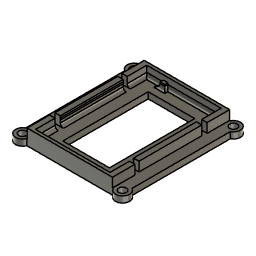
meanwell_holder v3 (Autodesk Fusion 360 design; units mm, degrees)
Autodesk Fusion 360 part; units mm, degrees
note: some values were not read from the file. Chosen so that the rebuilt part matches the saved one: which bodies a step acts on.
sketch "Sketch1" plane through (0, 0, 0) normal (0, 0, 1) x (1, 0, 0)
  line L0 (-23.5, 35.315) -> (23.5, 35.315)
  line L1 (23.5, 35.315) -> (23.5, -35.315)
  line L2 (23.5, -35.315) -> (-23.5, -35.315)
  line L3 (-23.5, -35.315) -> (-23.5, 35.315)
  line L4 (-23.5, 35.315) -> (23.5, -35.315) construction
  line L5 (23.5, 35.315) -> (-23.5, -35.315) construction
  circle A0 centre (-32, 35.75) radius 2.5
  circle A1 centre (32, 35.75) radius 2.5
  circle A2 centre (-31.9851, -36.25) radius 2.5
  circle A3 centre (32.0129, -35.7484) radius 2.5
  line L6 (-32, 35.75) -> (-30.3326, 33.8872) construction
  arc A4 (-34, -32.2263) -> (-27.7424, -37.75) centre (-31.9851, -36.25) ccw
  arc A5 (27.9826, -37.75) -> (34, -31.7109) centre (32.0129, -35.7484) ccw
  line L7 (-23.5, 26.2539) -> (28.9987, -32.397) construction
  arc A6 (34, 31.7189) -> (27.9689, 37.75) centre (32, 35.75) ccw
  line L8 (23.5, 26.2539) -> (-28.9987, -32.397) construction
  arc A7 (-27.9689, 37.75) -> (-34, 31.7189) centre (-32, 35.75) ccw
  line L9 (0, 35.75) -> (0, -35.75)
  line L10 (-34.0004, 29.5655) -> (-34.0155, -30.0752)
  line L11 (-25.6605, -37.75) -> (25.8288, -37.75)
  line L12 (34, -29.5596) -> (34, 29.5653)
  line L13 (25.8153, 37.75) -> (-25.8153, 37.75)
  line L14 (27.9689, 37.75) -> (-27.9689, 37.75)
  line L15 (25.8153, 37.75) -> (27.9689, 37.75)
  line L16 (34, 29.5653) -> (34, 31.7189)
  line L17 (34, -31.7109) -> (34, 31.7189)
  line L18 (-34, 31.7189) -> (-34, -32.2263)
  line L19 (-34, -37.7299) -> (-34, -37.75)
  line L20 (-34, -37.75) -> (-33.9851, -37.75)
  line L21 (-27.7424, -37.75) -> (27.9826, -37.75)
  dimension "d1" = 47
  dimension "d2" = 70.63
  dimension "d3" = 64
  dimension "d5" = 5
  dimension "d6" = 5
  dimension "d7" = 5
  dimension "d8" = 5
  dimension "d9" = 9
  dimension "d10" = 9
  dimension "d11" = 9
  dimension "d12" = 9
  dimension "d13" = 71.5
  constraint horizontal L0
  constraint perpendicular L0 L1
  constraint parallel L0 L2
  constraint parallel L1 L3
  constraint coincident L4 origin
  constraint coincident L5 origin
  constraint coincident origin L6
  constraint coincident A0.centre L6.start
  constraint concentric A1 A6
  constraint concentric A3 A5
  constraint concentric A2 A4
  constraint coincident A0 L6.end
  constraint collinear L6 L7
  constraint coincident L3 L7.start
  constraint coincident L1 L8.start
  constraint midpoint origin L9
  constraint horizontal L15
  constraint perpendicular L15 L16
  constraint horizontal L20
  constraint coincident A4.end L20
  constraint collinear L18 L19
  constraint coincident A2 L19.start
  constraint coincident A2 L20.end
  constraint collinear L20 L21
  measures "d1" distance of L1.end L2.end
  measures "d2" distance of L0.end L1.end
  measures "d3" distance of A2.centre A3.centre
  measures "d5" diameter of A0
  measures "d6" diameter of A1
  measures "d7" diameter of A2
  measures "d8" diameter of A3
  measures "d9" diameter of A6
  measures "d10" diameter of A5
  measures "d11" diameter of A4
  measures "d12" diameter of A7
  measures "d13" distance of L9.start L9.end
extrude "Extrude1" add sketch "Sketch1" along normal blind 4 contours L0 L2 L3 L9 | L0 L1 L2 L9 | A4 A5 A6 A7 L11 L12 L13 L14 L15 L16 L17 L18 L21 makes body 1
sketch "Sketch2" plane through (0, 0, 4) normal (0, 0, 1) x (-1, 0, 0)
  circle A0 centre (-32, -35.75) radius 2.5
  circle A1 centre (-32.0129, 35.7484) radius 2.5
  line L0 (33.9851, 37.75) -> (34, 37.75)
  line L1 (34, 37.75) -> (34, 37.7299)
  arc A2 (33.9851, 37.75) -> (34, 37.7299) centre (31.9851, 36.25) ccw
  circle A3 centre (32, -35.75) radius 2.5
  line L2 (-27.9689, -37.75) -> (27.9689, -37.75)
  arc A4 (27.9689, -37.75) -> (34, -31.7189) centre (32, -35.75) ccw
  line L3 (34, -31.7189) -> (34, 32.2263)
  arc A5 (34, 32.2263) -> (27.7424, 37.75) centre (31.9851, 36.25) ccw
  line L4 (27.7424, 37.75) -> (-27.9826, 37.75)
  arc A6 (-27.9826, 37.75) -> (-34, 31.7109) centre (-32.0129, 35.7484) ccw
  line L5 (-34, 31.7109) -> (-34, -31.7189)
  arc A7 (-34, -31.7189) -> (-27.9689, -37.75) centre (-32, -35.75) ccw
  line L6 (23.5, -35.315) -> (-23.5, -35.315)
  line L7 (23.5, 35.315) -> (23.5, -35.315)
  line L8 (-23.5, -35.315) -> (-23.5, 35.315)
  line L9 (-23.5, 35.315) -> (23.5, 35.315)
  line L10 (24, 32.815) -> (24, -35.815)
  line L11 (-25.5, 37.315) -> (25.5, 37.315)
  line L12 (25.5, 37.315) -> (25.5, -37.315)
  line L13 (25.5, -37.315) -> (-25.5, -37.315)
  line L14 (-25.5, -37.315) -> (-25.5, 37.315)
  line L15 (21, 35.815) -> (24, 32.815)
  line L16 (-21, 35.815) -> (-24, 32.815)
  line L17 (23.5, 35.315) -> (8.8, 35.315)
  line L18 (5.8, 33.815) -> (8.8, 33.815)
  line L19 (8.8, 33.815) -> (8.8, 35.815)
  line L20 (5.8, 36.815) -> (5.8, 33.815)
  line L21 (-8, 33.815) -> (-5, 33.815)
  line L22 (-5, 33.815) -> (-5, 35.815)
  line L23 (-8, 35.815) -> (-8, 33.815)
  line L24 (8.8, 35.815) -> (21, 35.815)
  line L25 (-21, 35.815) -> (-7, 35.815)
  line L26 (-5, 35.815) -> (6.8, 35.815)
  line L27 (23.5, 35.315) -> (8.8, 35.315)
  line L28 (5.8, 35.315) -> (-5, 35.315)
  line L29 (-21, -35.815) -> (-24, -32.815)
  line L30 (-23.5, -35.315) -> (10.4, -35.315)
  line L31 (13.4, -35.815) -> (13.4, -33.815)
  line L32 (13.4, -33.815) -> (10.4, -33.815)
  line L33 (10.4, -33.815) -> (10.4, -35.815)
  line L34 (10.4, -35.815) -> (-21, -35.815)
  line L35 (24, -35.815) -> (13.4, -35.815)
  line L36 (-23.5, -35.315) -> (-23.5, -15.615)
  line L37 (-22, -15.615) -> (-24, -15.615)
  line L38 (-24, -12.615) -> (-22, -12.615)
  line L39 (-22, -12.615) -> (-22, -15.615)
  line L40 (-24, -32.815) -> (-24, -15.615)
  line L41 (-24, -12.615) -> (-24, 32.815)
  line L42 (25.5, -37.75) -> (-25.5, -37.75)
  line L43 (-25.5, -37.75) -> (-25.5, 37.75)
  line L44 (-25.5, 37.75) -> (25.5, 37.75)
  line L45 (25.5, 37.75) -> (25.5, -37.75)
  point P0 (-24, 35.815)
  point P1 (24, 35.815)
  point P2 (-24, -35.815)
  point P3 (7.3, 35.315)
  point P4 (-6.5, 35.315)
  point P5 (-23.5, -14.115)
  dimension "d20" = -2
  dimension "d21" = 3
  dimension "d22" = 3
  dimension "d23" = 3
  dimension "d24" = 3
  dimension "d25" = 16.2
  dimension "d26" = 30
  dimension "d31" = 3
  dimension "d32" = 3
  dimension "d34" = 3
  dimension "d36" = 21.2
  constraint coincident P1 L25
  constraint coincident P1 L10
  constraint coincident P0 L25
  constraint coincident P0 L40
  constraint coincident L7.start L9.end
  constraint perpendicular L7 L17
  constraint perpendicular L7 L27
  constraint horizontal L18
  constraint perpendicular L18 L19
  constraint parallel L19 L20
  constraint horizontal L21
  constraint perpendicular L21 L22
  constraint parallel L22 L23
  constraint coincident L19.end L25
  constraint collinear L24 L25
  constraint coincident L22.end L25
  constraint coincident L23.start L25
  constraint collinear L25 L26
  constraint coincident L22 L28.end
  constraint coincident L20 L28.start
  constraint collinear L27 L28
  constraint coincident L19 L17.end
  constraint coincident P2 L35
  constraint coincident P2 L40
  constraint coincident L6.end L8.start
  constraint perpendicular L12 L30
  constraint parallel L31 L33
  constraint coincident L33.end L35
  constraint collinear L34 L35
  constraint coincident L33 L30.end
  constraint perpendicular L30 L36
  constraint horizontal L37
  constraint parallel L37 L38
  constraint coincident L38.start L40
  constraint collinear L40 L41
  constraint coincident L37 L36.end
  constraint horizontal L42
  constraint vertical L43
  constraint horizontal L44
  constraint vertical L45
  constraint coincident L4 L43.end
  constraint coincident L2 L42.start
  measures "d21" distance of P1 L15.start
  measures "d22" distance of P1 L10.start
  measures "d23" distance of P0 L16.start
  measures "d24" distance of P0 L16.end
  measures "d25" distance of L7.start P3
  measures "d26" distance of L7.start P4
  measures "d31" distance of P2 L29.start
  measures "d32" distance of P2 L29.end
  measures "d34" distance of L31.end L32.end
  measures "d36" distance of L6.end P5
extrude "Extrude2" add sketch "Sketch2" along normal blind 3 contours L2 L13 L42 L43 L45 | L11 L12 L13 L14 L43 L45 | L4 L11 L43 L44 L45 | L6 L31 L32 L33 | L7 L9 L15 L17 L27 | L6 L8 L29 L30 L36 | L9 L18 L19 L20 | L8 L37 L38 L39 | L9 L21 L22 L23 | L8 L9 L16 bodies 1
sketch "Sketch3" plane through (0, 0, 7) normal (0, 0, 1) x (-1, 0, 0)
  line L0 (-22, -15.615) -> (-22, -12.615)
  line L1 (-22, -12.615) -> (-24, -12.615)
  line L2 (-24, -12.615) -> (-24, 32.815)
  line L3 (-24, 32.815) -> (-21, 35.815)
  line L4 (-21, 35.815) -> (-8, 35.815)
  line L5 (-8, 35.815) -> (-8, 33.815)
  line L6 (-8, 33.815) -> (-5, 33.815)
  line L7 (-5, 33.815) -> (-5, 35.815)
  line L8 (-5, 35.815) -> (5.8, 35.815)
  line L9 (5.8, 35.815) -> (5.8, 33.815)
  line L10 (5.8, 33.815) -> (8.8, 33.815)
  line L11 (8.8, 33.815) -> (8.8, 35.815)
  line L12 (8.8, 35.815) -> (21, 35.815)
  line L13 (21, 35.815) -> (24, 32.815)
  line L14 (24, 32.815) -> (24, -35.815)
  line L15 (24, -35.815) -> (13.4, -35.815)
  line L16 (13.4, -35.815) -> (13.4, -33.815)
  line L17 (13.4, -33.815) -> (10.4, -33.815)
  line L18 (10.4, -33.815) -> (10.4, -35.815)
  line L19 (10.4, -35.815) -> (-21, -35.815)
  line L20 (-21, -35.815) -> (-24, -32.815)
  line L21 (-24, -32.815) -> (-24, -15.615)
  line L22 (-24, -15.615) -> (-22, -15.615)
  line L23 (25.5, 37.75) -> (-25.5, 37.75)
  line L24 (-25.5, 37.75) -> (-25.5, -37.75)
  line L25 (-25.5, -37.75) -> (25.5, -37.75)
  line L26 (25.5, -37.75) -> (25.5, 37.75)
  line L27 (23.5, -35.315) -> (-23.5, -35.315)
  line L28 (23.5, 35.315) -> (23.5, -35.315)
  line L29 (-23.5, -35.315) -> (-23.5, 35.315)
  line L30 (-23.5, 35.315) -> (23.5, 35.315)
  line L31 (-24, 35.815) -> (24, 35.815)
  line L32 (24, 35.815) -> (24, -35.815)
  line L33 (24, -35.815) -> (-24, -35.815)
  line L34 (-24, -35.815) -> (-24, 35.815)
  dimension "d41" = -0.5
extrude "Extrude3" add sketch "Sketch3" along normal blind 3 bodies 1
sketch "Sketch4" plane through (0, -35.815, 0) normal (0, 1, 0) x (-1, 0, 0)
  line L0 (-21, 4) -> (-8, 4)
  line L1 (-8, 4) -> (-8, 7)
  line L2 (-8, 7) -> (-5, 7)
  line L3 (-5, 7) -> (-5, 4)
  line L4 (-5, 4) -> (5.8, 4)
  line L5 (5.8, 4) -> (5.8, 7)
  line L6 (5.8, 7) -> (8.8, 7)
  line L7 (8.8, 7) -> (8.8, 4)
  line L8 (8.8, 4) -> (21, 4)
  line L9 (21, 4) -> (21, 7)
  line L10 (21, 7) -> (24, 7)
  line L11 (24, 7) -> (24, 10)
  line L12 (24, 10) -> (-24, 10)
  line L13 (-24, 10) -> (-24, 7)
  line L14 (-24, 7) -> (-21, 7)
  line L15 (-21, 7) -> (-21, 4)
  line L16 (-24, 7) -> (-24, 7.6962)
  line L17 (-23.5981, 9.1962) -> (-22.4613, 11.1651)
  line L18 (-24, 8.5) -> (-20.9226, 8.5) construction
  line L19 (-24, 10) -> (-22.2313, 6.9366)
  line L20 (-24, 10) -> (-20.4627, 10) construction
  line L21 (-24, 10) -> (24, 10)
  line L22 (0, 10) -> (0, 2)
  arc A0 (-23.5981, 9.1962) -> (-24, 7.6962) centre (-21, 7.6962) ccw
  line L23 (-24, 10) -> (-24, 7)
  line L24 (24, 10) -> (24, 7)
  line L25 (24, 10) -> (22.2313, 6.9366)
  arc A1 (24, 7.6962) -> (23.5981, 9.1962) centre (21, 7.6962) ccw
  line L26 (23.5981, 9.1962) -> (22.4613, 11.1651)
  dimension "d44" = 1.5
  dimension "d45" = 60
  dimension "d46" = 60
  dimension "d47" = 3
  constraint coincident L13.end L14.start
  constraint coincident L13 L18.start
  constraint horizontal L18
  constraint horizontal L20
  constraint coincident L12.end L13.start
  constraint coincident L11.end L12.start
  constraint midpoint L21 L22.start
  constraint perpendicular L21 L22
  constraint coincident L18.start L17
  constraint coincident L18.start L16
  constraint tangent L17 A0
  constraint tangent L16 A0
  constraint symmetric L13.end L22 L10.end
  constraint symmetric L17.end L22 L26.end
  constraint symmetric L12.end L22 L11.end
  constraint symmetric L19.end L22 L25.end
  constraint symmetric L22 L17.start A1.end
  constraint symmetric L22 L16.end A1.start
  constraint symmetric L22 A0 A1
  constraint symmetric L22 L12.end L11.end
  measures "d44" distance of L13.end L18.start
  measures "d45" angle of L17 L18
  measures "d46" angle of L19 L20
  measures "d47" radius of A0
fillet "Fillet1" radius 2 1 faces at (0.9333, 4.205, 4) on bodies 1
extrude "Extrude7" add 1 faces at (25.5, -12.5833, 8) along direction (1, 0, 0) blind 2 on bodies 1 bodies 1
extrude "Extrude8" add 1 faces at (-25.5, 12.5833, 8) along direction (-1, 0, 0) blind 2 on bodies 1 bodies 1
sketch "Sketch5" plane through (0, 0, 4) normal (0, 0, 1) x (-1, 0, 0)
  line L0 (-27.5, 37.75) -> (-27.9826, 37.75)
  arc A0 (-27.9826, 37.75) -> (-34, 31.7109) centre (-32.0129, 35.7484) ccw
  line L1 (-34, 31.7109) -> (-34, -31.7189)
  arc A1 (-34, -31.7189) -> (-27.9689, -37.75) centre (-32, -35.75) ccw
  line L2 (-27.9689, -37.75) -> (-27.5, -37.75)
  circle A2 centre (-32.0129, 35.7484) radius 2.5
  circle A3 centre (-32, -35.75) radius 2.5
  line L3 (-38.0756, 37.75) -> (39, 37.75)
  line L4 (39, 37.75) -> (39, 34.75)
  line L5 (39, 34.75) -> (-38.0756, 34.75)
  line L6 (-38.0756, 34.75) -> (-38.0756, 37.75)
  line L7 (39, 20.25) -> (-38.0756, 20.25)
  line L8 (-38.0756, 23.25) -> (39, 23.25)
  line L9 (-38.0756, 20.25) -> (-38.0756, 23.25)
  line L10 (39, 23.25) -> (39, 20.25)
  line L11 (39, 5.75) -> (-38.0756, 5.75)
  line L12 (-38.0756, 8.75) -> (39, 8.75)
  line L13 (-38.0756, 5.75) -> (-38.0756, 8.75)
  line L14 (39, 8.75) -> (39, 5.75)
  line L15 (39, -8.75) -> (-38.0756, -8.75)
  line L16 (-38.0756, -5.75) -> (39, -5.75)
  line L17 (-38.0756, -8.75) -> (-38.0756, -5.75)
  line L18 (39, -5.75) -> (39, -8.75)
  line L19 (39, -23.25) -> (-38.0756, -23.25)
  line L20 (-38.0756, -20.25) -> (39, -20.25)
  line L21 (-38.0756, -23.25) -> (-38.0756, -20.25)
  line L22 (39, -20.25) -> (39, -23.25)
  line L23 (39, -37.75) -> (-38.0756, -37.75)
  line L24 (-38.0756, -34.75) -> (39, -34.75)
  line L25 (-38.0756, -37.75) -> (-38.0756, -34.75)
  line L26 (39, -34.75) -> (39, -37.75)
  line L27 (-27.5, -37.75) -> (-27.5, 37.75)
  dimension "d54" = 3
  dimension "d57" = 0
  dimension "d58" = -72.5
  constraint horizontal L3
  constraint vertical L4
  constraint horizontal L5
  constraint vertical L6
  measures "d54" distance of L3.start L5.end
extrude "Extrude5" cut sketch "Sketch5" along normal blind 32.11 contours L1 L7 L8 L27 | L7 L8 L10 L27 | L1 L19 L20 L27 | L19 L20 L22 L27 bodies 1
sketch "Sketch6" plane through (0, 0, 4) normal (0, 0, 1) x (-1, 0, 0)
  line L0 (-27.5, 20.25) -> (-22, 20.25)
  line L1 (-22, -20.25) -> (-27.5, -20.25)
  line L2 (-27.5, 37.75) -> (-27.9826, 37.75)
  arc A0 (-27.9826, 37.75) -> (-34, 31.7109) centre (-32.0129, 35.7484) ccw
  line L3 (-34, 31.7109) -> (-34, -31.7189)
  arc A1 (-34, -31.7189) -> (-27.9689, -37.75) centre (-32, -35.75) ccw
  line L4 (-27.9689, -37.75) -> (-27.5, -37.75)
  line L5 (-27.5, -23.25) -> (-22, -23.25)
  line L6 (-22, -23.25) -> (-22, -31.9866)
  line L7 (-22, -31.9866) -> (-20.1716, -33.815)
  line L8 (-20.1716, -33.815) -> (8.4, -33.815)
  line L9 (8.4, -33.815) -> (8.4, -31.815)
  line L10 (8.4, -31.815) -> (15.4, -31.815)
  line L11 (15.4, -31.815) -> (15.4, -33.815)
  line L12 (15.4, -33.815) -> (22, -33.815)
  line L13 (22, -33.815) -> (22, -23.25)
  arc A2 (27.9689, -37.75) -> (34, -31.7189) centre (32, -35.75) ccw
  line L14 (34, -31.7189) -> (34, 32.2263)
  arc A3 (34, 32.2263) -> (27.7424, 37.75) centre (31.9851, 36.25) ccw
  line L15 (27.7424, 37.75) -> (27.5, 37.75)
  line L16 (27.5, 23.25) -> (22, 23.25)
  line L17 (22, 23.25) -> (22, 31.9866)
  line L18 (22, 31.9866) -> (20.1716, 33.815)
  line L19 (20.1716, 33.815) -> (10.8, 33.815)
  line L20 (10.8, 33.815) -> (10.8, 31.815)
  line L21 (10.8, 31.815) -> (3.8, 31.815)
  line L22 (3.8, 31.815) -> (3.8, 33.815)
  line L23 (3.8, 33.815) -> (-3, 33.815)
  line L24 (-3, 33.815) -> (-3, 31.815)
  line L25 (-3, 31.815) -> (-10, 31.815)
  line L26 (-10, 31.815) -> (-10, 33.815)
  line L27 (-10, 33.815) -> (-20.1716, 33.815)
  line L28 (-20.1716, 33.815) -> (-22, 31.9866)
  line L29 (-22, 31.9866) -> (-22, 23.25)
  line L30 (22, -20.25) -> (22, 20.25)
  line L31 (33.9851, 37.75) -> (34, 37.75)
  line L32 (34, 37.75) -> (34, 37.7299)
  arc A4 (33.9851, 37.75) -> (34, 37.7299) centre (31.9851, 36.25) ccw
  circle A5 centre (32, -35.75) radius 2.5
  circle A6 centre (-32, -35.75) radius 2.5
  line L33 (-22, 20.25) -> (-22, -10.615)
  line L34 (-22, -10.615) -> (-20, -10.615)
  line L35 (-20, -10.615) -> (-20, -17.615)
  line L36 (-20, -17.615) -> (-22, -17.615)
  line L37 (-22, -17.615) -> (-22, -20.25)
  circle A7 centre (-32.0129, 35.7484) radius 2.5
  line L38 (-15.2733, 27.5) -> (14.7267, 27.5)
  line L39 (14.7267, 27.5) -> (14.7267, -27.5)
  line L40 (14.7267, -27.5) -> (-15.2733, -27.5)
  line L41 (-15.2733, -27.5) -> (-15.2733, 27.5)
  line L42 (-15.2733, 27.5) -> (14.7267, -27.5) construction
  line L43 (14.7267, 27.5) -> (-15.2733, -27.5) construction
  line L44 (22, 20.25) -> (27.5, 20.25)
  line L45 (27.5, 20.25) -> (27.5, -20.25)
  line L46 (-27.5, 23.25) -> (-27.5, 37.75)
  line L47 (-27.5, -37.75) -> (-27.5, -23.25)
  line L48 (22, -23.25) -> (27.5, -23.25)
  line L49 (27.5, -23.25) -> (27.5, -37.75)
  line L50 (27.5, -37.75) -> (27.9689, -37.75)
  line L51 (27.5, 37.75) -> (27.5, 23.25)
  line L52 (-22, 23.25) -> (-27.5, 23.25)
  line L53 (-27.5, -20.25) -> (-27.5, 20.25)
  line L54 (27.5, -20.25) -> (22, -20.25)
  point P0 (-0.2733, 0)
  dimension "d61" = 30
  dimension "d62" = 55
  constraint horizontal L38
  constraint perpendicular L38 L39
  constraint parallel L38 L40
  constraint parallel L39 L41
  constraint coincident L42 P0
  constraint coincident L43 P0
  measures "d61" distance of L39.end L40.end
  measures "d62" distance of L38.end L39.end
extrude "Extrude6" cut sketch "Sketch6" against normal blind 9.662 contours L38 L39 L40 L41 bodies 1
extrude "Extrude4" add sketch "Sketch4" along normal blind 40.505 from surface at 15.56 contours L13 L17 L19 A0 L23 | L11 L24 L25 A1 L26 bodies 1
split "Split1" by plane through (0, 0, 4) normal (0, 0, 1) bodies 1 makes body 2 at (27.5, -6.75, 6) makes body 3 at (9.1667, 37.75, 8) makes body 4 at (9.1667, -37.75, 8) makes body 5 at (-27.5, 6.75, 6)
move_body "Move1" bodies 2 to x (1, 0, 0) y (0, 1, 0) z (0, 0, 1) at (-0.4, 0, 0)
move_body "Move2" bodies 5 to x (1, 0, 0) y (0, 1, 0) z (0, 0, 1) at (0.4, 0, 0)
combine "Combine1" operation add target body 1 tool bodies 2 5 4 3
equation "d22 = d21"
equation "d24 = d23"
equation "d32 = d31"
